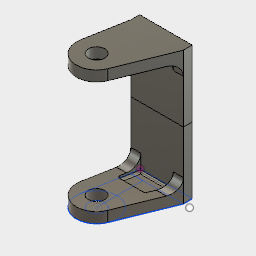
servo_bracket_ankle_2 (Autodesk Fusion 360 design; units mm, degrees)
Autodesk Fusion 360 part; units mm, degrees
note: some values were not read from the file. Set by a fixed rule: which sketch regions a step uses.
sketch "スケッチ1" plane through (0, 0, 0) normal (0, 1, 0) x (1, 0, 0)
  line L0 (0, 0) -> (13, 0)
  line L1 (13, 0) -> (13, -2.2)
  line L2 (13, -2.2) -> (0, -2.2)
  line L3 (0, -2.2) -> (0, 0)
  line L4 (0, -2.2) -> (3, -2.2)
  line L5 (3, -2.2) -> (3, -13.6)
  line L6 (3, -2.2) -> (14.4, -2.2) construction
  circle A0 centre (3, -13.6) radius 5
  circle A1 centre (3, -13.6) radius 2
  line L7 (0, -2.2) -> (-1.9186, -12.7014)
  line L8 (13, -2.2) -> (7.6357, -15.4735)
  dimension "d1" = 2.2
  dimension "d2" = 13
  dimension "d3" = 3
  dimension "d4" = 90
  dimension "d5" = 11.4
  dimension "d6" = 10
  dimension "d7" = 4
  measures "d1" distance of L0.start L2.end
  measures "d2" distance of L0.start L0.end
  measures "d3" distance of L2.end L4.end
  measures "d4" angle of L5 L6
  measures "d5" distance of L4.end L5.end
  measures "d6" diameter of A0
  measures "d7" diameter of A1
extrude "押し出し1" add sketch "スケッチ1" along normal blind 2.6 contours L2 L4 L5 A0 L7 | L2 L5 A0 L8 | A0 makes body 1
extrude "押し出し2" add sketch "スケッチ1" along normal blind 16.425 contours L0 L1 L2 L3 L4 bodies 1
fillet "フィレット1" radius 3 1 edges at (6.5, 2.6, 2.2) on bodies 1
ref_plane "作業平面1" through (6.5, 16.425, 1.1) normal (0, 1, 0) x (0, 0, 1)
delete_face "面を削除1" 1 faces at (7.8804, 2.6711, 4.5507) on bodies 1
sketch "スケッチ2" plane through (0, 2.6, 0) normal (0, 1, 0) x (-1, 0, 0)
  line L0 (-13, 2.2) -> (0, 2.2)
  line L1 (0, 2.2) -> (1.9186, 12.7014)
  arc A0 (1.9186, 12.7014) -> (-7.6357, 15.4735) centre (-3, 13.6) ccw
  line L2 (-7.6357, 15.4735) -> (-13, 2.2)
  circle A1 centre (-3, 13.6) radius 2
  line L3 (-10.5, 2.2) -> (-2.5, 2.2)
  line L4 (-2.5, 2.2) -> (-1.5865, 7.2)
  line L5 (-1.5865, 7.2) -> (-8.4793, 7.2)
  line L6 (-8.4793, 7.2) -> (-10.5, 2.2)
  dimension "d15" = 2.5
  dimension "d16" = 8
  dimension "d17" = 5
  measures "d15" distance of L0.start L3.start
  measures "d16" distance of L3.start L3.end
  measures "d17" distance of L3 L5
extrude "押し出し3" cut sketch "スケッチ2" against normal blind 1 contours L0 L3 L4 L5 L6 bodies 1
fillet "フィレット2" radius 3 2 edges at (1.25, 2.6, 2.2) (11.75, 2.6, 2.2) on bodies 1
fillet "フィレット3" radius 0.5 6 edges at (6.5, 1.6, 2.2) (2.0433, 1.6, 4.7) (5.0329, 1.6, 7.2) (1.5865, 2.1, 7.2) (8.4793, 2.1, 7.2) (9.4897, 1.6, 4.7) on bodies 1
mirror "ミラー2" about plane through (6.5, 16.425, 1.1) normal (0, 1, 0) of bodies 1 makes body 2
named bodies: "ボディ2"
